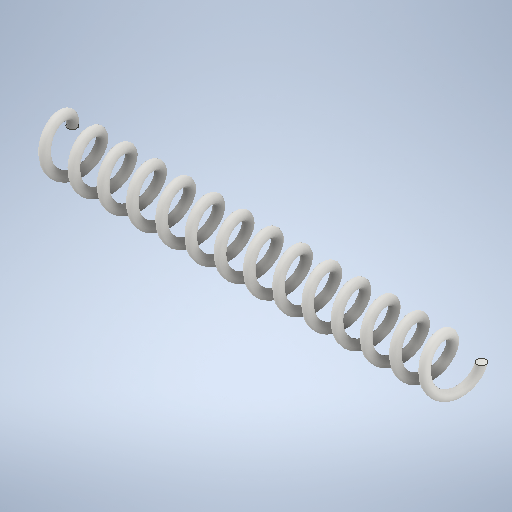
# Autodesk Inventor part: 9Sprężyna
Saved by Autodesk Inventor 2025 (Build 290162000, 162)
## iProperties
Created: 2025-03-22
Part Number: 9Sprężyna
Material: Stal kuta
Document SubType Name: Modeling
Designer: barte
Density: 7.85 g/cm^3
Appearance: Stal
Author: barte
Autodesk Inventor part; units mm, degrees
ref_plane "YZ Plane" through (0, 0, 0) normal (1, 0, 0) x (0, 1, 0)
ref_plane "XZ Plane" through (0, 0, 0) normal (0, 1, 0) x (-1, 0, 0)
ref_plane "XY Plane" through (0, 0, 0) normal (0, 0, 1) x (1, 0, 0)
sketch "Szkic1" plane through (0, 0, 0) normal (0, 1, 0) x (-1, 0, 0)
  line L0 (0, 13.0197) -> (10, 13.0197)
  circle A0 centre (5, -0.5803) radius 3
  point P0 (0, 0)
  point P1 (5, 13.0197)
  dimension "d0" = 10
  dimension "d1" = 6
  dimension "d2" = 13.6
  constraints: 2 end point, 1 centre point, 1 horizontal, 1 midpoint
  measures "d0" distance of L0.start L0.end
  measures "d1" diameter of A0
  measures "d2" distance of A0.centre point (5, 13.02)
coil "Zwój1" sketch "Szkic1" operation add axis through (0, 0, 13.0197) along (-1, 0, 0) pitch 19 turns 14 hand right
